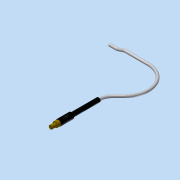
# Autodesk Inventor part: coax_tx
Saved by Autodesk Inventor 2014 SP1 (Build 180222100, 222)
## iProperties
Created: 2014-03-24
Part Number: coax_tx
Document SubType Name: Modeling
Designer: Robert Davis
Density: 1 g/cm^3
Material: Generic
Appearance: Default
Author: Robert Davis
Autodesk Inventor part; units mm, degrees
ref_plane "XZ Plane" through (0, 0, 0) normal (0, 1, 0) x (-1, 0, 0)
sketch "Sketch2" plane through (0, 0, 0) normal (0, 1, 0) x (-1, 0, 0)
  line L0 (0, 0) -> (-5, 0)
  line L1 (-5, 0) -> (-10, 1.6)
  line L2 (-10, 1.6) -> (-15, 1.6)
  dimension "d0" = 1.6
  dimension "d1" = 5
  dimension "d2" = 5
  dimension "d3" = 5
  constraints: 6 end point, 2 horizontal, 1 coincident
  measures "d0" distance between parallel lines of L0 L2
  measures "d1" distance of L0.start L0.end
  measures "d2" horizontal distance of L0.end L1.end
  measures "d3" distance of L1.end L2.end
sketch "Sketch3" plane through (0, 0, 0) normal (1, 0, 0) x (0, 1, 0)
  circle A0 centre (0, 0) radius 0.9
  dimension "d4" = 1.8
  constraints: 1 centre point, 1 coincident
  measures "d4" diameter of A0
sweep "Sweep1" add profiles "Sketch3" path "Sketch2"
ref_plane "Work Plane1" through (0, 0, 1.6) normal (0, 0, 1) x (1, 0, 0)
sketch "Sketch4" plane through (0, 0, 1.6) normal (0, 0, 1) x (1, 0, 0)
  line L0 (15, 0) -> (25, 0)
  line L1 (35.6066, -25.6066) -> (31.9289, -29.2843)
  line L2 (29, -36.3553) -> (29, -67.5)
  arc A0 (35.6066, -25.6066) -> (25, 0) centre (25, -15) ccw
  arc A1 (31.9289, -29.2843) -> (29, -36.3553) centre (39, -36.3553) ccw
  point P0 (0, 0)
  dimension "d7" = 15
  dimension "d8" = 15
  dimension "d9" = 10
  dimension "d10" = 10
  dimension "d11" = 45
  dimension "d13" = 14
  dimension "d14" = 67.5
  constraints: 6 end point, 4 point on circle, 4 tangent, 2 centre point, 1 horizontal, 1 point on line, 1 vertical
  measures "d7" distance of point (0, 0) L0.start
  measures "d8" radius of A0
  measures "d9" radius of A1
  measures "d10" distance of L0.start L0.end
  measures "d11" angle of L0 L1
  measures "d13" distance from line of L0.start L2
  measures "d14" distance from line of L2.end L0
ref_plane "Work Plane2" through (15, 0, 0) normal (1, 0, 0) x (0, 1, 0)
sketch "Sketch5" plane through (15, 0, 0) normal (1, 0, 0) x (0, 1, 0)
  circle A0 centre (0, 1.6) radius 0.9
  point P0 (0, 0)
  dimension "d16" = 1.6
  dimension "d17" = 1.8
  constraints: 1 centre point, 1 vertical alignment
  measures "d16" distance of point (0, 0) A0.centre
  measures "d17" diameter of A0
sweep "Sweep2" add profiles "Sketch5" path "Sketch4"
sketch "Sketch7" plane through (29, -67.5, 1.6) normal (0, -1, 0) x (1, 0, 0)
  circle A0 centre (0, 0) radius 0.9 projected
  circle A1 centre (0, 0) radius 1.2065
  point P0 (-29, -1.6)
  dimension "d21" = 2.413
  constraints: 1 centre point, 1 coincident
  measures "d21" diameter of A1
extrude "Extrusion1" add sketch "Sketch7" against normal blind 3.048
sketch "Sketch8" plane through (29, -64.452, 1.6) normal (0, 1, 0) x (1, 0, 0)
  circle A0 centre (0, 0) radius 0.9 projected
  circle A1 centre (0, 0) radius 1.2065 projected
  circle A2 centre (0, 0) radius 1.7526
  point P0 (-29, 1.6)
  dimension "d24" = 3.5052
  constraints: 1 centre point, 1 coincident
  measures "d24" diameter of A2
extrude "Extrusion2" add sketch "Sketch8" along normal blind 2.032 contours A1 | A2
sketch "Sketch9" plane through (29, -62.42, 1.6) normal (0, 1, 0) x (1, 0, 0)
  circle A0 centre (0, 0) radius 0.9 projected
  circle A1 centre (0, 0) radius 1.7526 projected
  circle A2 centre (0, 0) radius 1.905
  point P0 (-29, 1.6)
  dimension "d27" = 3.81
  constraints: 1 centre point, 1 coincident
  measures "d27" diameter of A2
extrude "Extrusion3" add sketch "Sketch9" along normal blind 8.382 contours A1 | A2
sketch "Sketch10" plane through (29, -54.038, 1.6) normal (0, 1, 0) x (1, 0, 0)
  circle A0 centre (0, 0) radius 0.9 projected
  circle A1 centre (0, 0) radius 1.905 projected
  circle A2 centre (0, 0) radius 1.3462
  point P0 (-29, 1.6)
  dimension "d30" = 2.6924
  constraints: 1 centre point, 1 coincident
  measures "d30" diameter of A2
extrude "Extrusion4" add sketch "Sketch10" along normal blind 17.78 contours A2
body "Solid1"
